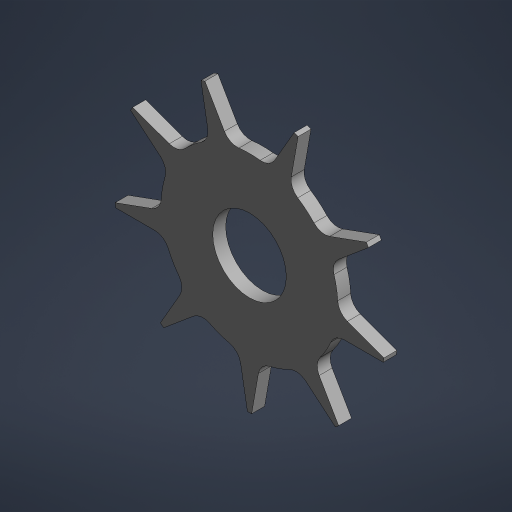
# Autodesk Inventor part: ROLLER,5
Saved by Autodesk Inventor 2023.4 (Build 274418000, 418)
## iProperties
Created: 2024-01-30
Part Number: ROLLER,5
Material: Generic
Document SubType Name: Modeling
Designer: john.thibert
Appearance: Default
Title: C:/Users/Jthib/OneDrive/Trifisk/CAD/Standard Parts/ROLLER/ROLLER,5.stp
Sending System: KeyCreator
Preprocessor: KCM Version 1.1.0.0
Autodesk Inventor part; units mm, degrees
ref_plane "YZ Plane" through (0, 0, 0) normal (1, 0, 0) x (0, 1, 0)
ref_plane "XZ Plane" through (0, 0, 0) normal (0, 1, 0) x (-1, 0, 0)
ref_plane "XY Plane" through (0, 0, 0) normal (0, 0, 1) x (1, 0, 0)
sketch "Sketch1" plane through (0, 0, 0) normal (0, 0, 1) x (1, 0, 0)
  line L0 (27.5881, 10.0556) -> (27.8558, 9.3368) construction
  line L1 (27.8558, 9.3368) -> (21.3609, 5.6433) construction
  arc A0 (21.3609, 5.6433) -> (19.6075, 2.6357) centre (22.5174, 2.9541) ccw construction
  arc A1 (19.529, -3.031) -> (19.6075, 2.6357) centre (-6.8308, 0.1684) ccw construction
  arc A2 (19.529, -3.031) -> (21.1242, -6.2153) centre (22.4904, -3.5391) ccw construction
  line L2 (27.6234, -9.961) -> (21.1242, -6.2153) construction
  line L3 (27.6234, -9.961) -> (27.3665, -10.6837) construction
  line L4 (14.515, -25.5221) -> (13.8537, -25.9105)
  circle A3 centre (0, 0) radius 7.9375
  circle A4 centre (0, 0) radius 29.3688
  point P0 (27.495, -10.3223)
  point P1 (27.722, 9.6962)
  dimension "d0" = 15.875
  dimension "d1" = 26.5532
  dimension "d2" = 58.7375
  constraints: 10 end point, 9 centre point, 8 point on circle, 3 coincident, 2 midpoint
  measures "d0" diameter of A3
  measures "d1" radius of A1
  measures "d2" diameter of A4
extrude "Extrusion1" add sketch "Sketch1" along normal blind 2.794
sketch "Sketch2" plane through (0, 0, 2.794) normal (0, 0, 1) x (1, 0, 0)
  line L0 (-9.6157, 27.75) -> (-5.4166, 20.4769)
  arc A0 (-5.4166, 20.4769) -> (-2.286, 18.9123) centre (-2.667, 22.0644) ccw
  arc A1 (2.286, 18.9123) -> (5.4166, 20.4769) centre (2.667, 22.0644) ccw
  line L1 (9.6157, 27.75) -> (5.4166, 20.4769)
  line L2 (0, 0) -> (0, 29.4775) construction
  arc A2 (2.286, 18.9123) -> (-2.286, 18.9123) centre (0, 0) ccw
  circle A3 centre (0, 0) radius 29.3687 projected
  dimension "d8" = 60
  dimension "d9" = 19.05
  dimension "d10" = 3.175
  dimension "d11" = 5.334
  constraints: 6 end point, 6 point on circle, 5 centre point, 3 coincident, 3 tangent, 1 vertical, 5 other
  measures "d8" angle of L1 L0
  measures "d9" radius of A2
  measures "d10" radius of A0
  measures "d11" distance of A1.centre A0.centre
extrude "Extrusion2" cut sketch "Sketch2" against normal through all contours A3 L1 A1 A2 A0 L0 picked at (0.2545, 25.8031)
pattern_circular "Circular Pattern1" count 9 over 360 about axis through (0, 0, 0) along (0, 0, 1) of "Extrusion2"
body "Solid1"
body "Solid7"
